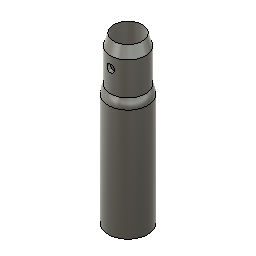
blindCoupler (Autodesk Fusion 360 design; units mm, degrees)
Autodesk Fusion 360 part; units mm, degrees
sketch "Sketch1" plane through (0, 0, 0) normal (0, 1, 0) x (1, 0, 0)
  circle A0 centre (0, 0) radius 7.5
  circle A1 centre (0, 0) radius 9
  circle A2 centre (-7.5, 0) radius 1.5
  circle A3 centre (0, -7.5) radius 1.5
  circle A4 centre (7.5, 0) radius 1.5
  circle A5 centre (0, 7.5) radius 1.5
  dimension "d1" = 15
  dimension "d2" = 1.5
  dimension "d3" = 3
  dimension "d5" = 360
  constraint coincident A0.centre A1.centre
  constraint coincident A0 A2.centre
  constraint horizontal A0.centre A2.centre
  measures "d1" diameter of A0
  measures "d3" diameter of A2
extrude "Extrude1" add sketch "Sketch1" along normal blind 55 contours A0 A4 | A0 A4 | A0 A1 A4 A5 | A0 A1 A3 A4 | A0 A5 | A0 A5 | A0 A3 | A0 A3 | A0 A1 A2 A5 | A0 A1 A2 A3 | A0 A2 | A0 A2
sketch "Sketch2" plane through (0, 55, 0) normal (0, 1, 0) x (-1, 0, 0)
  arc A0 (-7.35, -1.4925) -> (-7.35, 1.4925) centre (-7.5, 0) ccw
  arc A1 (-1.4925, 7.35) -> (-7.35, 1.4925) centre (0, 0) ccw
  arc A2 (-1.4925, 7.35) -> (1.4925, 7.35) centre (0, 7.5) ccw
  arc A3 (7.35, 1.4925) -> (1.4925, 7.35) centre (0, 0) ccw
  arc A4 (7.35, 1.4925) -> (7.35, -1.4925) centre (7.5, 0) ccw
  arc A5 (1.4925, -7.35) -> (7.35, -1.4925) centre (0, 0) ccw
  arc A6 (1.4925, -7.35) -> (-1.4925, -7.35) centre (0, -7.5) ccw
  arc A7 (-7.35, -1.4925) -> (-1.4925, -7.35) centre (0, 0) ccw
  circle A8 centre (0, 0) radius 9
  circle A9 centre (0, 0) radius 10.5
  circle A10 centre (0, 0) radius 6.5
  circle A11 centre (0, 0) radius 8
  dimension "d8" = 13
  dimension "d9" = 1.5
  constraint concentric A1 A9
  constraint coincident A1.centre A3.centre
  measures "d8" diameter of A10
extrude "Extrude2" add sketch "Sketch2" along normal blind 20 contours A0 A6 A7 A10 | A0 A1 A2 A10 | A4 A5 A6 A10 | A2 A3 A4 A10 | A11
fillet "Fillet1" radius 8.89 1 edges at (-8.3909, 55, 3.2545)
draft "Draft1" angle 1 neutral plane through (0, 0, 0) pull (0, -1, 0) 4 faces at (-7.2685, 36.6667, -1.8489) (-3.8664, 36.6667, 6.4266) (6.9214, 36.6667, 2.8885) (7.2685, 18.3333, -1.8489)
sketch "Sketch3" plane through (0, 0, 0) normal (1, 0, 0) x (0, 0, -1)
  circle A0 centre (0, 65) radius 1.75
  line L0 (8, 75) -> (-8, 75)
  dimension "d17" = 10
  dimension "d18" = 3.5
  measures "d17" distance of A0.centre L0
  measures "d18" diameter of A0
extrude "Extrude3" cut sketch "Sketch3" against normal blind 16
chamfer "Chamfer1" distance 1.5 distance2 5 1 edges at (7.4586, 75, -2.8929) measured on face at (-7.446, 75, -0.7204)
